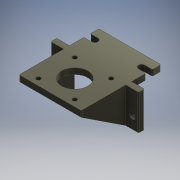
# Autodesk Inventor part: Z Motor Mount 1.0
Saved by Autodesk Inventor 2016 (Build 200138000, 138)
## iProperties
Created: 2017-02-10
Part Number: Z Motor Mount 1.0
Material: PC/ABS Plastic
Document SubType Name: Sheet Metal
Designer: Scott
Density: 0.357273 g/cm^3
Appearance: Gunmetal
Sheet Metal Rule: Default
Author: Scott
Autodesk Inventor part; units mm, degrees
ref_plane "YZ Plane" through (0, 0, 0) normal (1, 0, 0) x (0, 1, 0)
ref_plane "XZ Plane" through (0, 0, 0) normal (0, 1, 0) x (-1, 0, 0)
ref_plane "XY Plane" through (0, 0, 0) normal (0, 0, 1) x (1, 0, 0)
sketch "Sketch1" plane through (0, 0, 0) normal (0, 0, 1) x (1, 0, 0)
  circle A0 centre (0, 0) radius 11.2
  line L0 (-26.5, -21) -> (26.5, -21)
  line L1 (26.5, -21) -> (37.5, 17)
  line L2 (37.5, 17) -> (37.5, 47)
  line L3 (37.5, 47) -> (-37.5, 47)
  line L4 (-37.5, 47) -> (-37.5, 17)
  line L5 (-37.5, 17) -> (-26.5, -21)
  line L6 (-21.5, 24.7614) -> (-21.5, -34.1796) construction
  line L7 (21.5, 24.7614) -> (21.5, -37.8196) construction
  line L8 (-55.4202, 22) -> (54.2016, 22) construction
  dimension "d0" = 22.4
  dimension "d1" = 5
  dimension "d2" = 5
  dimension "d3" = 5
  dimension "d4" = 5
  dimension "d5" = 25
  dimension "d6" = 16
  dimension "d7" = 16
  dimension "d8" = 21.5
  dimension "d9" = 21.5
  dimension "d10" = 21
  dimension "d11" = 22
  constraints: 18 end point, 3 perpendicular, 2 horizontal, 2 vertical, 1 centre point, 1 coincident
  measures "d0" diameter of A0
  measures "d1" distance from line of L0.end L7
  measures "d2" distance from line of L6 L0.start
  measures "d3" distance from line of L1.end L8
  measures "d4" distance from line of L8 L4.end
  measures "d5" distance between parallel lines of L3 L8
  measures "d6" distance between parallel lines of L2 L7
  measures "d7" distance between parallel lines of L4 L6
  measures "d8" distance from line of A0.centre L6
  measures "d9" distance from line of A0.centre L7
  measures "d10" distance from line of L0 A0.centre
  measures "d11" distance from line of L8 A0.centre
extrude "Extrusion1" add sketch "Sketch1" along normal blind 5
sketch "Sketch2" plane through (0, 0, 0) normal (0, 0, -1) x (-1, 0, 0)
  line L0 (-26.5, -21) -> (-37.5, 17) projected
  line L1 (37.5, 17) -> (26.5, -21) projected
  line L2 (-26.5, -21) -> (-26.5, 17)
  line L3 (-26.5, 17) -> (-37.5, 17)
  line L4 (-37.5, 17) -> (-37.5, 47) projected
  line L5 (-37.5, 22) -> (-21.5, 22)
  line L6 (-21.5, 22) -> (-21.5, -21)
  line L7 (26.5, -21) -> (-26.5, -21) projected
  line L8 (-21.5, -21) -> (-26.5, -21)
  line L9 (26.5, -21) -> (26.5, 17)
  line L10 (26.5, 17) -> (37.5, 17)
  line L11 (37.5, 47) -> (37.5, 17) projected
  line L12 (37.5, 22) -> (21.5, 22)
  line L13 (21.5, 22) -> (21.5, -21)
  point P0 (0, 0)
  dimension "d14" = 5
  dimension "d15" = 5
  dimension "d16" = 5
  dimension "d17" = 5
  constraints: 18 end point, 6 perpendicular, 3 point on line, 2 horizontal, 1 vertical
  measures "d14" distance between parallel lines of L12 L10
  measures "d15" distance between parallel lines of L13 L9
  measures "d16" distance between parallel lines of L5 L3
  measures "d17" distance between parallel lines of L6 L2
extrude "Extrusion2" add sketch "Sketch2" along normal blind 25 contours L13 L12 L11 L10 L9 L7 | L2 L3 L4 L5 L6 L7
sketch "Sketch3" plane through (0, 0, 0) normal (1, 0, 0) x (0, 1, 0)
  line L0 (17, -25) -> (-21, -25) projected
  line L1 (-21, 0) -> (-21, -25) projected
  line L2 (-21, 0) -> (-21, -25) projected
  line L3 (-21, 0) -> (17, -25)
  line L4 (17, -25) -> (-21, -25)
  line L5 (-21, -25) -> (-21, 0)
  point P0 (0, 0)
  constraints: 6 end point, 1 horizontal
extrude "Extrusion3" cut sketch "Sketch3" along normal through all both and the other way through all
sketch "Sketch4" plane through (0, 0, 5) normal (0, 0, 1) x (1, 0, 0)
  line L0 (-37.5, 17) -> (-26.5, -21) projected
  line L1 (-37.5, 17) -> (-26.5, 17) projected
  line L2 (-26.5, 17) -> (-26.5, -21) projected
  line L3 (26.5, 17) -> (37.5, 17) projected
  line L4 (26.5, -21) -> (26.5, 17) projected
  line L5 (26.5, -21) -> (37.5, 17) projected
  line L6 (37.5, 22) -> (21.5, 22) projected
  line L7 (-21.5, 22) -> (-37.5, 22) projected
  line L8 (37.5, 47) -> (-37.5, 47) projected
  line L9 (-26.5, 17) -> (-26.5, -21) projected
  line L10 (-37.5, 17) -> (-26.5, -21)
  line L11 (-26.5, -21) -> (-26.5, 17)
  line L12 (-26.5, 17) -> (-37.5, 17) projected
  line L13 (-26.5, 17) -> (-37.5, 17)
  line L14 (37.5, 17) -> (26.5, 17) projected
  line L15 (26.5, 17) -> (37.5, 17)
  line L16 (37.5, 17) -> (26.5, -20)
  line L17 (26.5, -20) -> (26.5, 17)
  line L18 (-26.5, 22) -> (-26.5, 47)
  line L19 (37.5, 47) -> (-37.5, 47) projected
  line L20 (-26.5, 47) -> (-37.5, 47)
  line L21 (-37.5, 47) -> (-37.5, 22)
  line L22 (-37.5, 22) -> (-26.5, 22)
  line L23 (21.5, 22) -> (37.5, 22) projected
  line L24 (26.5, 22) -> (26.5, 47)
  line L25 (26.5, 47) -> (37.5, 47)
  line L26 (37.5, 22) -> (37.5, 17) projected
  line L27 (37.5, 47) -> (37.5, 22)
  line L28 (37.5, 22) -> (26.5, 22)
  point P0 (0, 0)
  constraints: 28 end point, 7 collinear, 6 perpendicular, 4 point on line, 1 horizontal
extrude "Extrusion4" cut sketch "Sketch4" against normal through all
sketch "Sketch5" plane through (0, 0, 5) normal (0, 0, 1) x (1, 0, 0)
  line L0 (0, 0) -> (0, 29.9357) construction
  line L1 (0, 0) -> (-35.6616, 0) construction
  line L2 (-15.5, 15.5) -> (15.5, 15.5) construction
  line L3 (15.5, 15.5) -> (15.5, -15.5) construction
  line L4 (15.5, -15.5) -> (-15.5, -15.5) construction
  line L5 (-15.5, -15.5) -> (-15.5, 15.5) construction
  point P0 (0, 15.5)
  point P1 (-15.5, 0)
  dimension "d24" = 31
  dimension "d25" = 31
  constraints: 12 end point, 4 coincident, 2 horizontal, 2 midpoint, 2 parallel, 2 point on line, 1 perpendicular, 1 vertical
  measures "d24" distance of L2.start L2.end
  measures "d25" distance of L2.end L3.end
hole "Hole1" at (-15.5, 15.5, 5) at (15.5, 15.5, 5) at (15.5, -15.5, 5) at (-15.5, -15.5, 5) direction (0, 0, -1) diameter 3.5 end through all
sketch "Sketch6" plane through (26.5, 17, 5) normal (0, -1, 0) x (1, 0, 0)
  line L0 (-48, -5) -> (-5, -5) projected
  line L1 (-53, -30) -> (-53, -5) projected
  line L2 (0, -5) -> (0, -30) projected
  line L3 (-84.7583, -20) -> (35.1169, -20) construction
  point P0 (-26.5, -5)
  point P1 (5.5, -20)
  point P2 (-58.5, -20)
  dimension "d33" = 15
  dimension "d34" = 5.5
  dimension "d35" = 5.5
  constraints: 2 end point, 2 point on line, 1 horizontal
  measures "d33" distance between parallel lines of L3 L0
  measures "d34" distance from line of L1 point (-58.5, -20)
  measures "d35" distance from line of L2 point (5.5, -20)
hole "Hole2" at (32, 17, -15) at (-32, 17, -15) direction (0, 1, 0) diameter 5.4 end through all
sketch "Sketch7" plane through (0, 0, 5) normal (0, 0, 1) x (1, 0, 0)
  line L0 (-26.0966, 37) -> (27.6353, 37) construction
  line L1 (-30, 37) -> (-20, 37)
  line L2 (-30, 34.3) -> (-20, 34.3)
  line L3 (-20, 39.7) -> (-30, 39.7)
  arc A0 (-30, 39.7) -> (-30, 34.3) centre (-30, 37) ccw
  arc A1 (-20, 34.3) -> (-20, 39.7) centre (-20, 37) ccw
  line L4 (20, 37) -> (30, 37)
  line L5 (20, 34.3) -> (30, 34.3)
  line L6 (30, 39.7) -> (20, 39.7)
  arc A2 (20, 39.7) -> (20, 34.3) centre (20, 37) ccw
  arc A3 (30, 34.3) -> (30, 39.7) centre (30, 37) ccw
  line L7 (-26.5, 22) -> (-37.5, 22) construction
  point P0 (0, 0)
  point P1 (-25, 37)
  point P2 (25, 37)
  dimension "d43" = 5.4
  dimension "d44" = 15
  dimension "d46" = 20
  dimension "d47" = 20
  dimension "d48" = 10
  dimension "d49" = 10
  constraints: 18 end point, 8 point on circle, 8 tangent, 4 centre point, 4 point on line, 2 midpoint, 2 parallel, 1 collinear, 1 horizontal
  measures "d43" distance between parallel lines of L5 L6
  measures "d44" distance between parallel lines of L7 L0
  measures "d46" horizontal distance of point (0, 0) L1.end
  measures "d47" horizontal distance of L4.start point (0, 0)
  measures "d48" distance of L1.start L1.end
  measures "d49" distance of L4.end L4.start
extrude "Extrusion5" cut sketch "Sketch7" against normal through all
fillet "Fillet1" radius 1 1 edges at (37.5, 17, -10)
fillet "Fillet2" radius 1 13 edges at (37.5, 22, -10) (26.5, 34.3, 2.5) (26.5, 39.7, 2.5) (26.5, 47, 2.5) (-26.5, 47, 2.5) (-26.5, 39.7, 2.5) (-26.5, 34.3, 2.5) (-37.5, 22, -10) (-37.5, 17, -10) (-26.5, -21, 2.5) (-21.5, 22, -12.5) (21.5, 22, -12.5) (26.5, -21, 2.5)
equation "\"BendRadius\" = Thickness"
equation "\"BendReliefWidth\" = Thickness"
equation "\"BendReliefDepth\" = 0.5 * Thickness"
equation "\"CornerReliefSize\" = 4 * Thickness"
equation "\"MinimumRemnant\" = 2 * Thickness"
equation "\"TransitionRadius\" = BendRadius"
equation "\"JacobiRadiusSize\" = Thickness"
equation "\"GapSize\" = Thickness"
equation "\"Thickness\" = 0.5"
body "Solid1"
